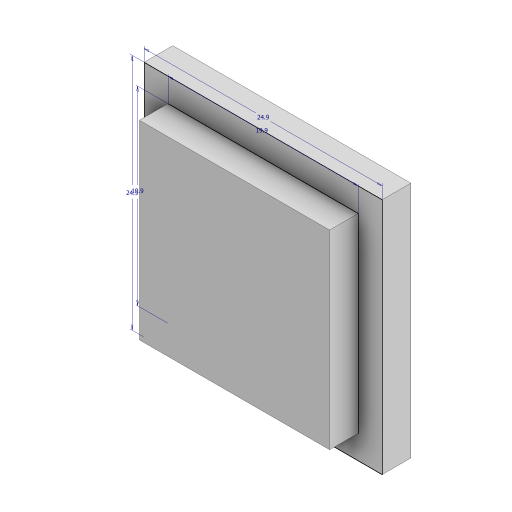
# Autodesk Inventor part: Large-cuvette-cap-25mm
Saved by Autodesk Inventor 2023 (Build 270158000, 158)
## iProperties
Created: 2023-04-14
Part Number: Large-cuvette-cap-25mm
Material: Generic
Document SubType Name: Modeling
Designer: nvladi
Density: 1 g/cm^3
Appearance: Default
Author: nvladi
Autodesk Inventor part; units mm, degrees
ref_plane "YZ Plane" through (0, 0, 0) normal (1, 0, 0) x (0, 1, 0)
ref_plane "XZ Plane" through (0, 0, 0) normal (0, 1, 0) x (-1, 0, 0)
ref_plane "XY Plane" through (0, 0, 0) normal (0, 0, 1) x (1, 0, 0)
sketch "Sketch1" plane through (0, 0, 0) normal (0, 0, 1) x (1, 0, 0)
  line L0 (9.95, -9.95) -> (-9.95, -9.95)
  line L1 (-9.95, -9.95) -> (-9.95, 9.95)
  line L2 (-9.95, 9.95) -> (9.95, 9.95)
  line L3 (9.95, 9.95) -> (9.95, -9.95)
  line L4 (12.45, -12.45) -> (-12.45, -12.45)
  line L5 (-12.45, -12.45) -> (-12.45, 12.45)
  line L6 (-12.45, 12.45) -> (12.45, 12.45)
  line L7 (12.45, 12.45) -> (12.45, -12.45)
  dimension "d2" = 19.9
  dimension "d3" = 19.9
  dimension "d5" = 24.9
  dimension "d6" = 24.9
  constraints: 16 end point, 4 parallel, 2 horizontal, 2 perpendicular
  measures "d2" distance between parallel lines of L3 L1
  measures "d3" distance between parallel lines of L0 L2
  measures "d5" distance of L5.end L6.end
  measures "d6" distance of L4.end L5.end
extrude "Extrusion1" add sketch "Sketch1" along normal blind 3 contours L0 L1 L2 L3
extrude "Extrusion2" add sketch "Sketch1" against normal blind 3 contours L0 L1 L2 L3 | L4 L5 L6 L7
body "Solid1"
